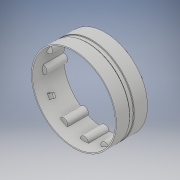
# Autodesk Inventor part: than
Saved by Autodesk Inventor 2019 (Build 230136000, 136)
## iProperties
Created: 2021-01-08
Part Number: than
Material: Generic
Document SubType Name: Modeling
Designer: Admin
Density: 1 g/cm^3
Appearance: Default
Author: Admin
Autodesk Inventor part; units mm, degrees
ref_plane "YZ Plane" through (0, 0, 0) normal (1, 0, 0) x (0, 1, 0)
sketch "Sketch1" plane through (0, 0, 0) normal (0, 0, 1) x (1, 0, 0)
  circle A0 centre (0, 0) radius 200
  circle A1 centre (0, 0) radius 205
  line L0 (0, 0) -> (0, 200)
  line L1 (0, 0) -> (173.2051, -100)
  line L2 (-173.2051, -100) -> (0, 0)
  arc A2 (82.2012, 182.3265) -> (116.7988, 162.3516) centre (100, 173.2051) ccw
  arc A3 (162.3516, 116.7988) -> (182.3265, 82.2012) centre (173.2051, 100) ccw
  arc A4 (199, 19.975) -> (199, -19.975) centre (200, 0) ccw
  arc A5 (116.7988, -162.3516) -> (82.2012, -182.3265) centre (100, -173.2051) ccw
  arc A6 (19.975, -199) -> (-19.975, -199) centre (0, -200) ccw
  arc A7 (-82.2012, -182.3265) -> (-116.7988, -162.3516) centre (-100, -173.2051) ccw
  arc A8 (-199, -19.975) -> (-199, 19.975) centre (-200, 0) ccw
  arc A9 (-182.3265, 82.2012) -> (-162.3516, 116.7988) centre (-173.2051, 100) ccw
  arc A10 (-116.7988, 162.3516) -> (-82.2012, 182.3265) centre (-100, 173.2051) ccw
  dimension "d0" = 400
  dimension "d1" = 410
  dimension "d2" = 120
  dimension "d3" = 120
  constraints: 18 point on circle, 10 centre point, 6 end point, 2 coincident, 1 vertical, 23 other
  measures "d1" diameter of A1
  measures "d2" angle of L1 L0
  measures "d3" angle of L1 L2
extrude "Extrusion1" add sketch "Sketch1" along normal blind 150
extrude "Extrusion2" add sketch "Sketch1" along normal blind 100 contours A0 A4 | A3 A0 | A0 A5 | A2 A0 | A0 A6 | A10 A0 | A0 A8 | A7 A0 | A9 A0
ref_plane "Work Plane1" through (173.2051, 100, 100) normal (0, 0, 1) x (1, 0, 0)
sketch "Sketch2" plane through (173.2051, 100, 100) normal (0, 0, 1) x (1, 0, 0)
  arc A0 (-372.2051, -119.975) -> (-290.0039, -262.3516) centre (-173.2051, -100) ccw projected
  line L0 (-324.7595, -187.5) -> (-319.7595, -196.1603)
  line L1 (-319.7595, -196.1603) -> (-341.4102, -208.6603)
  line L2 (-341.4102, -208.6603) -> (-346.4102, -200)
  line L3 (-324.7595, -187.5) -> (-329.7595, -178.8397)
  line L4 (-329.7595, -178.8397) -> (-351.4102, -191.3397)
  line L5 (-351.4102, -191.3397) -> (-346.4102, -200)
  line L6 (-21.6506, -187.5) -> (-16.6506, -178.8397)
  line L7 (-16.6506, -178.8397) -> (5, -191.3397)
  line L8 (5, -191.3397) -> (0, -200)
  line L9 (-21.6506, -187.5) -> (-26.6506, -196.1603)
  line L10 (-26.6506, -196.1603) -> (-5, -208.6603)
  line L11 (-5, -208.6603) -> (0, -200)
  dimension "d19" = 25
  dimension "d20" = 10
  dimension "d21" = 25
  dimension "d22" = 10
  constraints: 24 end point, 2 parallel, 1 point on circle
  measures "d19" distance of L2.end L0.start
  measures "d20" distance of L0.start L0.end
  measures "d21" distance of L8.end L6.start
  measures "d22" distance of L6.start L6.end
extrude "Extrusion3" add sketch "Sketch2" against normal blind 10
fillet "Fillet1" radius 2 1 edges at (-167.9884, -108.5352, 95)
fillet "Fillet2" radius 2 1 edges at (-177.9884, -91.2147, 95)
fillet "Fillet3" radius 2 2 edges at (167.9884, -108.5352, 95) (177.9884, -91.2147, 95)
ref_plane "Work Plane2" through (0, 0, 75) normal (0, 0, 1) x (1, 0, 0)
sketch "Sketch3" plane through (0, 0, 75) normal (0, 0, 1) x (1, 0, 0)
  circle A0 centre (0, 0) radius 205
  circle A1 centre (0, 0) radius 202.5
  dimension "d28" = 405
  constraints: 2 centre point, 2 coincident
  measures "d28" diameter of A1
extrude "Extrusion4" cut sketch "Sketch3" along normal mid plane 20
fillet "Fillet4" radius 2 4 edges at (-202.5, 0, 85) (-205, 0, 85) (-202.5, 0, 65) (-205, 0, 65)
sketch "Sketch6" plane through (0, 0, 0) normal (0, 0, -1) x (-1, 0, 0)
  line L0 (0, -200) -> (-5, -200)
  line L1 (-5, -200) -> (-5, -195)
  line L2 (-5, -195) -> (0, -195)
  line L3 (0, -200) -> (5, -200)
  line L4 (5, -200) -> (5, -195)
  line L5 (5, -195) -> (0, -195)
  line L6 (100, -173.2051) -> (95.6699, -175.7051)
  line L7 (95.6699, -175.7051) -> (93.1699, -171.375)
  line L8 (93.1699, -171.375) -> (97.5, -168.875)
  line L9 (100, -173.2051) -> (104.3301, -170.7051)
  line L10 (104.3301, -170.7051) -> (101.8301, -166.375)
  line L11 (101.8301, -166.375) -> (97.5, -168.875)
  line L12 (173.2051, -100) -> (170.7051, -104.3301)
  line L13 (170.7051, -104.3301) -> (166.375, -101.8301)
  line L14 (166.375, -101.8301) -> (168.875, -97.5)
  line L15 (173.2051, -100) -> (175.7051, -95.6699)
  line L16 (175.7051, -95.6699) -> (171.375, -93.1699)
  line L17 (171.375, -93.1699) -> (168.875, -97.5)
  line L18 (200, 0) -> (200, -5)
  line L19 (200, -5) -> (195, -5)
  line L20 (195, -5) -> (195, 0)
  line L21 (200, 0) -> (200, 5)
  line L22 (200, 5) -> (195, 5)
  line L23 (195, 5) -> (195, 0)
  line L24 (173.2051, 100) -> (175.7051, 95.6699)
  line L25 (175.7051, 95.6699) -> (171.375, 93.1699)
  line L26 (171.375, 93.1699) -> (168.875, 97.5)
  line L27 (173.2051, 100) -> (170.7051, 104.3301)
  line L28 (170.7051, 104.3301) -> (166.375, 101.8301)
  line L29 (166.375, 101.8301) -> (168.875, 97.5)
  line L30 (100, 173.2051) -> (104.3301, 170.7051)
  line L31 (104.3301, 170.7051) -> (101.8301, 166.375)
  line L32 (101.8301, 166.375) -> (97.5, 168.875)
  line L33 (100, 173.2051) -> (95.6699, 175.7051)
  line L34 (95.6699, 175.7051) -> (93.1699, 171.375)
  line L35 (93.1699, 171.375) -> (97.5, 168.875)
  line L36 (0, 200) -> (5, 200)
  line L37 (5, 200) -> (5, 195)
  line L38 (5, 195) -> (0, 195)
  line L39 (0, 200) -> (-5, 200)
  line L40 (-5, 200) -> (-5, 195)
  line L41 (-5, 195) -> (0, 195)
  line L42 (-100, 173.2051) -> (-95.6699, 175.7051)
  line L43 (-95.6699, 175.7051) -> (-93.1699, 171.375)
  line L44 (-93.1699, 171.375) -> (-97.5, 168.875)
  line L45 (-100, 173.2051) -> (-104.3301, 170.7051)
  line L46 (-104.3301, 170.7051) -> (-101.8301, 166.375)
  line L47 (-101.8301, 166.375) -> (-97.5, 168.875)
  line L48 (-173.2051, 100) -> (-170.7051, 104.3301)
  line L49 (-170.7051, 104.3301) -> (-166.375, 101.8301)
  line L50 (-166.375, 101.8301) -> (-168.875, 97.5)
  line L51 (-173.2051, 100) -> (-175.7051, 95.6699)
  line L52 (-175.7051, 95.6699) -> (-171.375, 93.1699)
  line L53 (-171.375, 93.1699) -> (-168.875, 97.5)
  line L54 (-200, 0) -> (-200, 5)
  line L55 (-200, 5) -> (-195, 5)
  line L56 (-195, 5) -> (-195, 0)
  line L57 (-200, 0) -> (-200, -5)
  line L58 (-200, -5) -> (-195, -5)
  line L59 (-195, -5) -> (-195, 0)
  line L60 (-173.2051, -100) -> (-175.7051, -95.6699)
  line L61 (-175.7051, -95.6699) -> (-171.375, -93.1699)
  line L62 (-171.375, -93.1699) -> (-168.875, -97.5)
  line L63 (-173.2051, -100) -> (-170.7051, -104.3301)
  line L64 (-170.7051, -104.3301) -> (-166.375, -101.8301)
  line L65 (-166.375, -101.8301) -> (-168.875, -97.5)
  line L66 (-100, -173.2051) -> (-104.3301, -170.7051)
  line L67 (-104.3301, -170.7051) -> (-101.8301, -166.375)
  line L68 (-101.8301, -166.375) -> (-97.5, -168.875)
  line L69 (-100, -173.2051) -> (-95.6699, -175.7051)
  line L70 (-95.6699, -175.7051) -> (-93.1699, -171.375)
  line L71 (-93.1699, -171.375) -> (-97.5, -168.875)
  point P0 (0, 0)
  point P1 (0, 0)
  dimension "d34" = 360
  constraints: 144 end point, 1 coincident, 1 horizontal, 1 parallel, 1 perpendicular, 145 other
extrude "Extrusion5" add sketch "Sketch6" along normal blind 5 contours L0 L1 L2 L5 L4 L3 | L6 L7 L8 L11 L10 L9 | L18 L19 L20 L23 L22 L21 | L24 L25 L26 L29 L28 L27 | L30 L31 L32 L35 L34 L33 | L42 L43 L44 L47 L46 L45 | L48 L49 L50 L53 L52 L51 | L54 L55 L56 L59 L58 L57 | L66 L67 L68 L71 L70 L69
body "Solid1"
